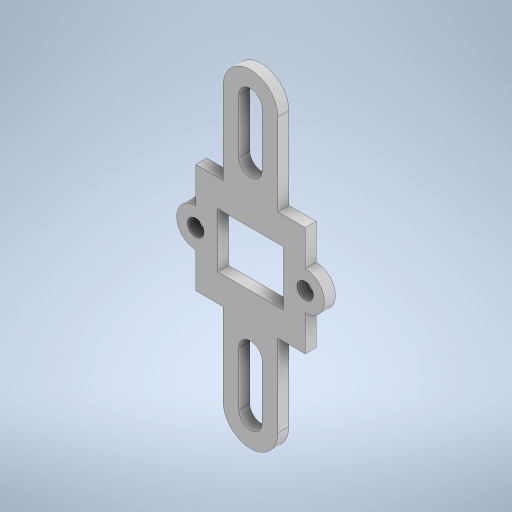
# Autodesk Inventor part: Time of Flight Attachment
Saved by Autodesk Inventor 2024 (Build 280153000, 153)
## iProperties
Created: 2023-10-25
Part Number: Time of Flight Attachment
Material: Generic
Document SubType Name: Modeling
Designer: olson
Density: 1 g/cm^3
Appearance: Default
Author: olson
Autodesk Inventor part; units mm, degrees
ref_plane "YZ Plane" through (0, 0, 0) normal (1, 0, 0) x (0, 1, 0)
ref_plane "XZ Plane" through (0, 0, 0) normal (0, 1, 0) x (-1, 0, 0)
ref_plane "XY Plane" through (0, 0, 0) normal (0, 0, 1) x (1, 0, 0)
sketch "Sketch1" plane through (0, 0, 0) normal (0, 0, 1) x (1, 0, 0)
  line L0 (0, 0) -> (10, 0)
  line L1 (0, 0) -> (-10, 0)
  line L2 (-10, 0) -> (-10, -6.5)
  line L3 (10, 0) -> (10, -6.5)
  line L4 (-10, 0) -> (10, 0)
  line L5 (-10, -20) -> (10, -20)
  line L6 (-10, -6.5) -> (-10, -5)
  line L7 (-6, -5) -> (6, -5)
  line L8 (-6, -15) -> (6, -15)
  line L9 (6, -5) -> (6, -15)
  line L10 (-6, -5) -> (-6, -15)
  line L11 (-10, 0) -> (-10, -6.5)
  line L12 (-10, -13.5) -> (-10, -20)
  line L13 (10, -20) -> (10, -13.5)
  line L14 (10, -6.5) -> (10, 0)
  circle A0 centre (10, -10) radius 1.5
  arc A1 (10, -13.5) -> (10, -6.5) centre (10, -10) ccw
  circle A2 centre (-10, -10) radius 1.5
  arc A3 (-10, -6.5) -> (-10, -13.5) centre (-10, -10) ccw
  dimension "d0" = 10
  dimension "d1" = 10
  dimension "d2" = 20
  dimension "d7" = 3
  dimension "d8" = 7
  dimension "d9" = 3
  dimension "d10" = 7
  constraints: 30 end point, 8 perpendicular, 4 centre point, 4 point on circle, 2 coincident, 2 horizontal, 1 parallel, 1 point on line
  measures "d0" distance of L0.start L0.end
  measures "d1" distance of L0.start L1.end
  measures "d2" distance of L1.end L5.start
  measures "d7" diameter of A0
  measures "d8" diameter of A1
  measures "d9" diameter of A2
  measures "d10" diameter of A3
extrude "Extrusion1" add sketch "Sketch1" along normal blind 2
thread "Thread2" size "M3x0.5" class "6H" standard "ANSI Metric M Profile" full length
thread "Thread3" size "M3x0.5" class "6H" standard "ANSI Metric M Profile" full length
sketch "Sketch6" plane through (0, 0, 2) normal (0, 0, 1) x (1, 0, 0)
  line L0 (10, 0) -> (-10, 0) projected
  line L1 (-5, 0) -> (-5, 20)
  line L2 (-5, 0) -> (15, 0) construction
  line L3 (-5, 20) -> (5, 20)
  line L4 (5, 20) -> (5, 0)
  arc A0 (-10, -6.5) -> (-10, -13.5) centre (-10, -10) ccw projected
  arc A1 (10, -13.5) -> (10, -6.5) centre (10, -10) ccw projected
  line L5 (0, 20) -> (0, 9.84)
  circle A2 centre (0, 14.92) radius 2.125
  line L6 (0, 0) -> (0, 10.16)
  circle A3 centre (0, 5.08) radius 2.125
  line L7 (-2.125, 14.92) -> (-2.125, 5.08)
  line L8 (2.125, 14.92) -> (2.125, 5.08)
  line L9 (-13.5, -10) -> (13.5, -10)
  line L10 (10, -20) -> (-10, -20)
  line L11 (-5, -20) -> (-5, -40)
  line L12 (-5, -40) -> (5, -40)
  line L13 (5, -40) -> (5, -20)
  line L14 (0, -40) -> (0, -29.84)
  circle A4 centre (0, -34.92) radius 2.125
  line L15 (0, -20) -> (0, -30.16)
  circle A5 centre (0, -25.08) radius 2.125
  line L16 (-2.125, -34.92) -> (-2.125, -25.08)
  line L17 (2.125, -34.92) -> (2.125, -25.08)
  dimension "d45" = 20
  dimension "d47" = 10
  dimension "d52" = 10.16
  dimension "d53" = 4.25
  dimension "d54" = 10.16
  dimension "d55" = 4.25
  constraints: 34 end point, 16 symmetric about line, 10 point on circle, 6 point on line, 4 centre point, 4 perpendicular, 3 midpoint, 2 tangent, 1 horizontal, 1 vertical, 2 other
  measures "d45" distance of L1.start L1.end
  measures "d47" distance of L1.end L3.end
  measures "d52" distance of L5.start L5.end
  measures "d53" diameter of A2
  measures "d54" distance of L6.start L6.end
  measures "d55" diameter of A3
extrude "Extrusion7" add sketch "Sketch6" against normal blind 2 contours L0 L6 A3 L8 A2 L5 L3 L4 | L0 L1 L3 L5 A2 L7 A3 L6 | L13 L12 L14 A4 L17 A5 L15 L10 | L15 A5 L16 A4 L14 L12 L11 L10
fillet "Fillet2" radius 5 4 edges at (5, -40, 1) (-5, -40, 1) (5, 20, 1) (-5, 20, 1)
body "Solid1"
